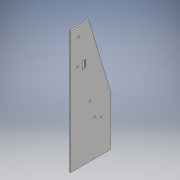
# Autodesk Inventor part: Part1
Saved by Autodesk Inventor 2018 (Build 220112000, 112)
## iProperties
Created: 2018-07-05
Part Number: Part1
Material: 一般
Document SubType Name: Modeling
Designer: KITformula
Density: 1 g/cm^3
Appearance: 既定
Author: KITformula
Autodesk Inventor part; units mm, degrees
ref_plane "YZ Plane" through (0, 0, 0) normal (1, 0, 0) x (0, 1, 0)
ref_plane "XZ Plane" through (0, 0, 0) normal (0, 1, 0) x (-1, 0, 0)
ref_plane "XY Plane" through (0, 0, 0) normal (0, 0, 1) x (1, 0, 0)
sketch "スケッチ1" plane through (0, 0, 0) normal (1, 0, 0) x (0, 1, 0)
  line L0 (0, 268.5) -> (0, -268.5)
  line L1 (0, -268.5) -> (175, -268.5)
  line L2 (175, -268.5) -> (175, -48.1515)
  line L3 (175, -48.1515) -> (80, 268.5)
  line L4 (80, 268.5) -> (0, 268.5)
  circle A0 centre (35.142, 228.391) radius 4.1
  circle A1 centre (30.426, 117.793) radius 4.1
  circle A2 centre (83.157, -37.222) radius 3.05
  circle A3 centre (104.738, -109.112) radius 3.05
  circle A4 centre (133.242, -123.706) radius 3.05
  line L5 (65, 128.5) -> (50, 128.5)
  line L6 (50, 128.5) -> (50, 98.5)
  line L7 (50, 98.5) -> (65, 98.5)
  line L8 (65, 98.5) -> (65, 128.5)
  point P0 (0, 0)
  point P1 (0, 0)
  dimension "d0" = 537
  dimension "d1" = 175
  dimension "d2" = 80
  dimension "d3" = 16.7
  dimension "d4" = 40.109
  dimension "d5" = 35.142
  dimension "d6" = 8.2
  dimension "d7" = 150.707
  dimension "d8" = 30.426
  dimension "d9" = 8.2
  dimension "d10" = 305.722
  dimension "d11" = 83.157
  dimension "d12" = 377.612
  dimension "d13" = 104.738
  dimension "d14" = 6.1
  dimension "d15" = 6.1
  dimension "d16" = 133.242
  dimension "d17" = 392.206
  dimension "d18" = 6.1
  dimension "d19" = 140
  dimension "d20" = 50
  dimension "d21" = 30
  dimension "d22" = 15
  constraints: 18 end point, 5 centre point, 3 parallel, 3 perpendicular, 1 coincident, 1 horizontal, 1 midpoint, 1 vertical
  measures "d0" distance of L0.start L0.end
  measures "d1" distance of L0.end L1.end
  measures "d2" distance of L3.end L0.start
  measures "d3" angle of L0 L3
  measures "d4" distance from line of L4 A0.centre
  measures "d5" distance from line of L0 A0.centre
  measures "d6" diameter of A0
  measures "d7" distance from line of L4 A1.centre
  measures "d8" distance from line of L0 A1.centre
  measures "d9" diameter of A1
  measures "d10" distance from line of L4 A2.centre
  measures "d11" distance from line of L0 A2.centre
  measures "d12" distance from line of L4 A3.centre
  measures "d13" distance from line of L0 A3.centre
  measures "d14" diameter of A2
  measures "d15" diameter of A3
  measures "d16" distance from line of L0 A4.centre
  measures "d17" distance from line of L4 A4.centre
  measures "d18" diameter of A4
  measures "d19" distance from line of L4 L5.end
  measures "d20" distance between parallel lines of L0 L6
  measures "d21" distance of L7.end L5.start
  measures "d22" distance of L5.start L5.end
extrude "押し出し1" add sketch "スケッチ1" along normal blind 5
